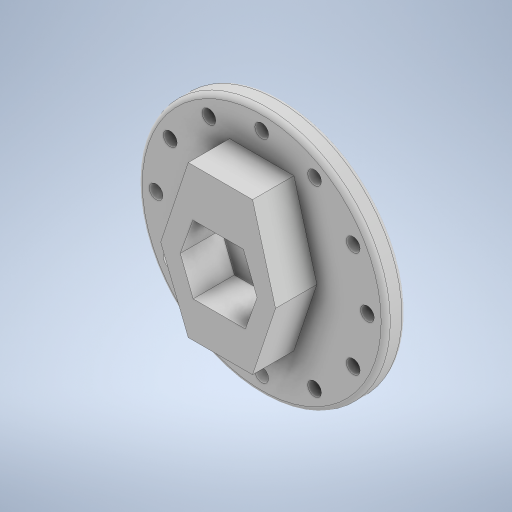
# Autodesk Inventor part: 1-26
Saved by Autodesk Inventor 2024.2 (Build 282272000, 272)
## iProperties
Created: 2024-11-02
Part Number: 1-26
Material: Generic
Document SubType Name: Modeling
Designer: Jimena Brenes
Density: 1 g/cm^3
Appearance: Default
Author: Jimena Brenes
Autodesk Inventor part; units mm, degrees
ref_plane "YZ Plane" through (0, 0, 0) normal (1, 0, 0) x (0, 1, 0)
ref_plane "XZ Plane" through (0, 0, 0) normal (0, 1, 0) x (-1, 0, 0)
ref_plane "XY Plane" through (0, 0, 0) normal (0, 0, 1) x (1, 0, 0)
sketch "Sketch1" plane through (0, 0, 0) normal (0, 0, 1) x (1, 0, 0)
  arc A0 (-8.2462, 16) -> (8.2462, 16) centre (0, 0) ccw
  line L0 (-8.2462, 16) -> (8.2462, 16)
  dimension "d0" = 36
  dimension "d1" = 16
  constraints: 2 end point, 2 point on circle, 1 centre point, 1 coincident, 1 horizontal
  measures "d0" diameter of A0
  measures "d1" distance from line of A0.centre L0
extrude "Extrusion1" add sketch "Sketch1" along normal blind 2
sketch "Sketch2" plane through (0, 0, 2) normal (0, 0, 1) x (1, 0, 0)
  circle A0 centre (0, 0) radius 27
  circle A1 centre (0, 0) radius 23 construction
  line L0 (0, 27) -> (0, -27) construction
  line L1 (-27, 0) -> (27, 0) construction
  line L2 (8.2462, 16) -> (-8.2462, 16) projected
  line L3 (8.2462, 16) -> (-8.2462, 16) projected
  arc A2 (-8.2462, 16) -> (8.2462, 16) centre (0, 0) ccw projected
  circle A3 centre (0, 23) radius 1.5
  circle A4 centre (11.5, 19.9186) radius 1.5
  circle A5 centre (19.9186, 11.5) radius 1.5
  circle A6 centre (23, 0) radius 1.5
  circle A7 centre (19.9186, -11.5) radius 1.5
  circle A8 centre (11.5, -19.9186) radius 1.5
  circle A9 centre (0, -23) radius 1.5
  circle A10 centre (-11.5, -19.9186) radius 1.5
  circle A11 centre (-19.9186, -11.5) radius 1.5
  circle A12 centre (-23, 0) radius 1.5
  circle A13 centre (-19.9186, 11.5) radius 1.5
  circle A14 centre (-11.5, 19.9186) radius 1.5
  dimension "d5" = 46
  dimension "d4" = 54
  dimension "d6" = 3
  dimension "d9" = 360
  constraints: 13 centre point, 4 end point, 4 point on circle, 2 coincident, 1 perpendicular, 1 vertical alignment, 27 other
  measures "d4" diameter of A0
  measures "d6" diameter of A3
extrude "Extrusion2" add sketch "Sketch2" along normal blind 4.5 contours A0 | A2 L2
chamfer "Chamfer1" distance 2 angle 45 1 edges at (0, 16, 0)
fillet "Fillet1" radius 1 2 edges at (-27, 0, 2) (-27, 0, 6.5)
sketch "Sketch3" plane through (0, 0, 0) normal (0, 0, -1) x (-1, 0, 0)
  circle A0 centre (0, 0) radius 7
  dimension "d17" = 14
  constraints: 1 centre point, 1 coincident
  measures "d17" diameter of A0
hole "Hole1" at (0, 0, 0) direction (0, 0, 1) diameter 8 end through all
sketch "Sketch4" plane through (0, 0, 6.5) normal (0, 0, 1) x (1, 0, 0)
  line L0 (0, 0) -> (0, 31) construction
  line L1 (-7, 18) -> (7, 18)
  line L2 (-7, 18) -> (-13, 0)
  line L3 (0, 0) -> (0, -27) construction
  line L4 (-7, -15) -> (7, -15)
  line L5 (-7, -15) -> (-13, 0)
  line L6 (7, 18) -> (12, 0)
  line L7 (12, 0) -> (7, -15)
  line L8 (-6, 7.6667) -> (5, 7.6667)
  line L9 (5, 7.6667) -> (8, 0)
  line L10 (8, 0) -> (5.4377, -7.1718)
  line L11 (5.4377, -7.1718) -> (-5.9328, -7.1718)
  line L12 (-5.9328, -7.1718) -> (-8.7391, 0)
  line L13 (-8.7391, 0) -> (-6, 7.6667)
  point P0 (0, 18)
  dimension "d27" = 14
  dimension "d28" = 14
  dimension "d31" = 11
  constraints: 28 end point, 3 parallel, 2 horizontal, 2 vertical, 1 coincident, 1 midpoint, 1 perpendicular, 1 point on line
  measures "d27" distance of L1.start L1.end
  measures "d28" distance of L4.start L4.end
  measures "d31" distance of L8.start L8.end
extrude "Extrusion4" add sketch "Sketch4" along normal blind 9
body "Solid1"
